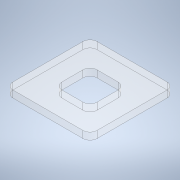
# Autodesk Inventor part: hot_glue_mashroom
Saved by Autodesk Inventor 2021 (Build 250183000, 183)
## iProperties
Created: 2022-02-27
Part Number: hot_glue_mashroom
Material: Generic
Document SubType Name: Modeling
Designer: ermoz
Density: 1 g/cm^3
Appearance: Default
Author: ermoz
Autodesk Inventor part; units mm, degrees
ref_plane "YZ Plane" through (0, 0, 0) normal (1, 0, 0) x (0, 1, 0)
ref_plane "XZ Plane" through (0, 0, 0) normal (0, 1, 0) x (-1, 0, 0)
ref_plane "XY Plane" through (0, 0, 0) normal (0, 0, 1) x (1, 0, 0)
sketch "Sketch1" plane through (0, 0, 0) normal (0, 1, 0) x (-1, 0, 0)
  line L0 (0, 0) -> (24, 0)
  line L1 (24, 0) -> (24, -24)
  line L2 (24, -24) -> (0, -24)
  line L3 (0, -24) -> (0, 0)
  dimension "d0" = 24
  dimension "d1" = 24
  constraints: 8 end point, 2 parallel, 1 horizontal, 1 perpendicular
  measures "d0" distance of L1.end L2.end
  measures "d1" distance of L0.end L1.end
extrude "Extrusion1" add sketch "Sketch1" along normal blind 2
sketch "Sketch2" plane through (0, 2, 0) normal (0, 1, 0) x (1, 0, 0)
  line L0 (0, 24) -> (-24, 24) projected
  line L1 (-24, 0) -> (0, 0) projected
  line L2 (-24, 24) -> (0, 0)
  line L3 (0, 24) -> (-24, 0)
  line L4 (-17, 17) -> (-7, 17)
  line L5 (-7, 17) -> (-7, 7)
  line L6 (-7, 7) -> (-17, 7)
  line L7 (-17, 7) -> (-17, 17)
  line L8 (-17, 17) -> (-7, 7) construction
  line L9 (-7, 17) -> (-17, 7) construction
  point P0 (-12, 12)
  point P1 (-12, 12)
  dimension "d4" = 10
  constraints: 16 end point, 5 midpoint, 2 parallel, 2 point on line, 1 horizontal, 1 perpendicular
  measures "d4" distance of L4.end L5.end
extrude "Extrusion2" cut sketch "Sketch2" against normal through all contours L5 L2 L3 | L3 L2 L4 | L2 L3 L7 | L2 L6 L3
fillet "Fillet1" radius 2 8 edges at (0, 1, 0) (0, 1, -24) (-24, 1, 0) (-24, 1, -24) (-7, 1, -17) (-17, 1, -17) (-17, 1, -7) (-7, 1, -7)
body "Solid1"
